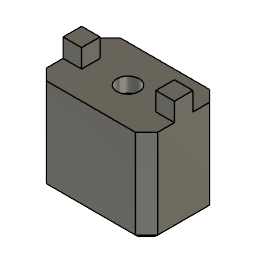
single leg (Autodesk Fusion 360 design; units mm, degrees)
Autodesk Fusion 360 part; units mm, degrees
note: some values were not read from the file. Set by a fixed rule: which sketch regions a step uses.
sketch "Szkic1" plane through (0, 0, 0) normal (0, 0, 1) x (1, 0, 0)
  line L0 (-15, 10) -> (15, 10)
  line L1 (15, 10) -> (15, -10)
  line L2 (15, -10) -> (-15, -10)
  line L3 (-15, -10) -> (-15, 10)
  circle A0 centre (0, 0) radius 3
  circle A1 centre (0, 0) radius 5.5
  line L4 (-15, 2.5) -> (-15, -2.5)
  line L5 (-15, -2.5) -> (15, -2.5)
  line L6 (15, -2.5) -> (15, 2.5)
  line L7 (15, 2.5) -> (-15, 2.5)
  line L8 (-10, 2.5) -> (10, 2.5)
  line L9 (10, 2.5) -> (10, -2.5)
  line L10 (10, -2.5) -> (-10, -2.5)
  line L11 (-10, -2.5) -> (-10, 2.5)
  dimension "d1" = 6
  dimension "d2" = 11
  constraint perpendicular L0 L1
  constraint parallel L0 L2
  constraint parallel L1 L3
  constraint horizontal L0
  constraint coincident A0.centre A1.centre
  constraint perpendicular L4 L5
  constraint parallel L4 L6
  constraint parallel L5 L7
  constraint coincident L3 L4.end
  constraint coincident L3 L4.start
  constraint perpendicular L8 L9
  constraint parallel L8 L10
  constraint parallel L9 L11
  constraint coincident L7 L8.end
  constraint parallel L7 L8
  measures "d1" diameter of A0
  measures "d2" diameter of A1
extrude "Wyciągnięcie proste1" add sketch "Szkic1" against normal blind 25 contours L0 L1 L3 A1 L7 L8 | L3 L4 L5 L7 L11 | L1 L5 L6 L7 L9 | L1 L2 L3 A1 L5 L10 | A1 L5 L7 L8 L10 L11 | A1 L5 L7 L8 L9 L10
extrude "Wyciągnięcie proste2" add sketch "Szkic1" against normal blind 4.2 contours A0 A1 L5 L7 L8 L10 | A0 A1 L7 L8 | A0 A1 L5 L7 L8 L10 | A0 A1 L5 L10 | A0 L5 L7 L8 L10 | A0 L7 L8 | A0 L5 L10
extrude "Wyciągnięcie proste3" cut sketch "Szkic1" against normal blind 4 contours A0 L5 L7 L8 L10 | A0 L7 L8 | A0 L5 L10
extrude "Wyciągnięcie proste4" add sketch "Szkic1" along normal blind 5 contours L3 L4 L5 L7 L11 | L1 L5 L6 L7 L9
chamfer "Fazowanie1" distance 3 angle 45 4 edges at (15, -10, -12.5) (15, 10, -12.5) (-15, -10, -12.5) (-15, 10, -12.5)
chamfer "Fazowanie2" distance 1 angle 45 1 faces at (11.8333, 0, -25)
delete_face "Usuń powierzchnię1" 1 faces at (6.159, 0.3074, -24.6667)
